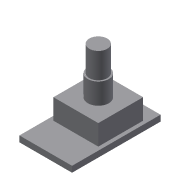
# Autodesk Inventor part: encoder
Saved by Autodesk Inventor 2020 (Build 240168000, 168)
## iProperties
Created: 2022-10-11
Part Number: encoder
Material: Allgemein
Document SubType Name: Modeling
Designer: uch10113
Density: 1 g/cm^3
Appearance: Vorgabe
Author: uch10113
Autodesk Inventor part; units mm, degrees
ref_plane "YZ Plane" through (0, 0, 0) normal (1, 0, 0) x (0, 1, 0)
ref_plane "XZ Plane" through (0, 0, 0) normal (0, 1, 0) x (-1, 0, 0)
ref_plane "XY Plane" through (0, 0, 0) normal (0, 0, 1) x (1, 0, 0)
sketch "Skizze1" plane through (0, 0, 0) normal (0, 0, 1) x (1, 0, 0)
  circle A0 centre (0, 0) radius 3.5
  dimension "d0" = 7
  constraints: 1 centre point, 1 coincident
  measures "d0" diameter of A0
extrude "Extrusion1" add sketch "Skizze1" along normal blind 7
sketch "Skizze2" plane through (0, 0, 0) normal (0, 0, -1) x (-1, 0, 0)
  line L0 (-7.5, 7.5) -> (7.5, 7.5)
  line L1 (7.5, 7.5) -> (7.5, -7.5)
  line L2 (7.5, -7.5) -> (-7.5, -7.5)
  line L3 (-7.5, -7.5) -> (-7.5, 7.5)
  line L4 (-7.5, 7.5) -> (7.5, -7.5) construction
  line L5 (7.5, 7.5) -> (-7.5, -7.5) construction
  point P0 (0, 0)
  dimension "d3" = 15
  dimension "d4" = 15
  constraints: 12 end point, 2 midpoint, 2 parallel, 1 horizontal, 1 perpendicular
  measures "d3" distance of L0.end L1.end
  measures "d4" distance of L0.start L0.end
extrude "Extrusion2" add sketch "Skizze2" along normal blind 6.8
sketch "Skizze3" plane through (0, 0, -6.8) normal (0, 0, -1) x (-1, 0, 0)
  line L0 (-8.6809, 12.15) -> (8.9191, 12.15)
  line L1 (8.9191, 12.15) -> (8.9191, -17.45)
  line L2 (8.9191, -17.45) -> (-8.6809, -17.45)
  line L3 (-8.6809, -17.45) -> (-8.6809, 12.15)
  line L4 (7.5, 7.5) -> (-7.5, 7.5) projected
  point P0 (0, 0)
  dimension "d7" = 17.6
  dimension "d8" = 29.6
  dimension "d9" = 4.65
  constraints: 8 end point, 2 parallel, 1 horizontal, 1 perpendicular
  measures "d7" distance of L0.start L0.end
  measures "d8" distance of L0.end L1.end
  measures "d9" distance between parallel lines of L4 L0
extrude "Extrusion3" add sketch "Skizze3" along normal blind 2
sketch "Skizze4" plane through (0, 0, 7) normal (0, 0, 1) x (1, 0, 0)
  circle A0 centre (0, 0) radius 3
  dimension "d12" = 6
  constraints: 1 centre point, 1 coincident
  measures "d12" diameter of A0
extrude "Extrusion4" add sketch "Skizze4" along normal blind 13.5
sketch "Skizze5" plane through (0, 0, 20.5) normal (0, 0, 1) x (1, 0, 0)
  line L0 (-8.9965, 8.617) -> (9.175, 8.617)
  line L1 (9.175, 8.617) -> (9.175, -9.4653)
  line L2 (9.175, -9.4653) -> (-8.9965, -9.4653)
  line L3 (-8.9965, -9.4653) -> (-8.9965, 8.617)
  point P0 (0, 0)
  constraints: 8 end point, 2 parallel, 1 horizontal, 1 perpendicular
extrude "Extrusion5" cut sketch "Skizze5" against normal blind 5
equation "\"d4\" = d3"
